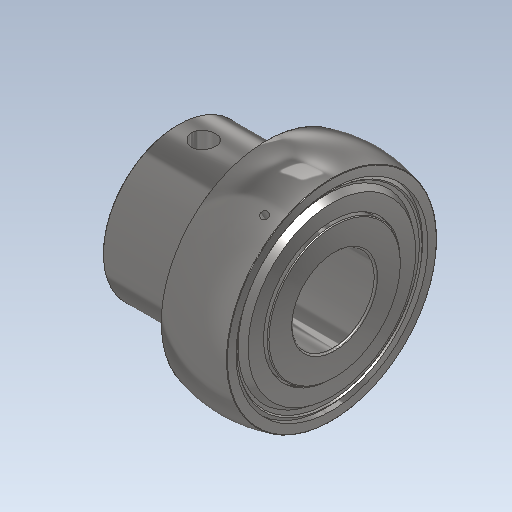
# Autodesk Inventor part: YET 203/15-24.21030112021228.6-bearing
Saved by Autodesk Inventor 2020 (Build 240168000, 168)
## iProperties
Part Number: YET 203/15-24.21030112021228.6-bearing
Material: Stainless Steel
Catalog Web Link: www.cadenas.de
Description: ayf_001hc_hh_hy_bearing-Y-bearings
Vendor: SKF
Document SubType Name: Modeling
Designer: partserver
Manufacturer: SKF
Mass: 107.476 g
Surface Area: 122.39 cm^2
Volume: 13.4345 cm^3
Density: 8 g/cm^3
Appearance: Semi-Polished
Category: PARTsolutions
Company: SKF
PSOL_IDENT_0: {$CADENAS_DATA\23d-libs\skf\bearings_units_and_housings\bearing_units\ball_bearing_units\y-units\y-b
PSOL_IDENT_1: earing_square_flanged_units_parts\ayf_001hc_hh_hy_bearing.prj},235 {VTYP=3D},{NB=YET 203/15-24.21030
PSOL_IDENT_2: 112021228.6-bearing},{LINA=YET 203/15-24.21030112021228.6-bearing},{NN=ayf_001hc_hh_hy_bearing},{DAT
PSOL_IDENT_3: E=20.08.2020 13:45:20},{GEOMDATE=29.07.2020 17:09:33},{VERSION=},{LINEID=2150},{WBVAR=},{WBNUMERIC=}
PSOL_IDENT_4: {NB=YET 203/15-24.21030112021228.6-bearing},{LINA=YET 203/15-24.21030112021228.6-bearing},{KT=DUMM
PSOL_IDENT_5: Y},{PRODUCTID=103011202},{DESIGNATION=YET 203/15},{DD=15.0000},{D=40},{B=19.100},{C=12.000},{PITCH=2
PSOL_IDENT_6: 8.500},{DW=6.747},{FO=IEC_BBY_005},{DESIGN=ybrg2},{B1=28.600},{LM=Eccentric locking collar},{DES=Inn
PSOL_IDENT_7: er ring extended on one side},{PS=For agricultural applications},{MAT=},{SS=Standard seals},{UNIT=Me
PSOL_IDENT_8: tric},{G=MIN},{DD1=24.20},{DD2=27.20},{DD3=MIN},{B3=13.500},{B4=4.8},{BB4=MIN},{R12=0.3},{R12X=0},{S
PSOL_IDENT_9: S1=22.100},{NOTE=},{DG=MIN},{E=3.600},{F=1.300},{RG=MIN},{LOAD1=9.560},{LOAD2=4.750},{LOAD3=0.200},{
PSOL_IDENT_10: SPEED2=9500},{FF0=13},{BF=1},{A15=500000},{A8=400000},{A4=300000},{BETA=1.89},{SBT1=0.094},{SBT2=},{
PSOL_IDENT_11: RF1=0.00000039},{RF2=1.7},{SF1=0.00323},{SF2=36.5},{KZ=3.1},{II=1},{Z=8},{SG=VT307},{MASS=0.12},{G2=
PSOL_IDENT_12: M6x0.75},{HEX=3.000},{RTT=4},{MKIT=},{AS=},{TANGLE=},{SLEEVE=},{SRING=RIS 203},{FPC=RBC17_YBRG_003},
PSOL_IDENT_13: {POPI=1},{NOUN=N020},{NOUNDES=Ball bearing},{MOD=M200},{MODDES=Radial deep groove},{YZ=12.1},{PIM=YE
PSOL_IDENT_14: T 203/15},{LNDD11=MIN},{LUB3=0},{BZ=0.3502},{SDALG=h},{YRZ=17.6235},{SHAPE=1},{LNB1HM11=0},{LWM=0},{
PSOL_IDENT_15: TYPEID=103011},{LUBGR2=0},{LOCKNUT=},{LOCKDEVICE=},{LNB=MIN},{BB=MIN},{LNB1=MIN},{S1ALG=0},{HH=MIN},
PSOL_IDENT_16: {LDB=MIN},{LDDD1=MIN},{LDDD2=MIN},{LDM=MIN},{LDFF=MIN},{TP=4},{LNBHM11=0},{BBHM11=0},{LNDD1HM11=0},{
PSOL_IDENT_17: HELP=3},{HHHM11=0},{LUBGR1=0},{LWV=0},{S2=0},{LUB2=1},{BZ1=0.000},{HEX2=}
NB: YET 203/15-24.21030112021228.6-bearing
NN: ayf_001hc_hh_hy_bearing
NT: Y-bearings
NBSYN: $DESIGNATION.-$DD1.$PRODUCTID.$C.$B1.-bearing
LINA: YET 203/15-24.21030112021228.6-bearing
CATALOG: SKF
DESIGNATION: YET 203/15
DD: 15
D: 40
B: 19.1
C: 12
B1: 28.6
DD1: 24.2
LOAD1: 9.56
LOAD2: 4.75
LOAD3: 0.2
SPEED2: 9500
SUPPLIER: SKF
ARTICLENO: YET 203/15-24.21030112021228.6-bearing
BOMINFO: YET 203/15-24.21030112021228.6-bearing
CREATOR: CADENAS GmbH
Title: YET 203/15-24.21030112021228.6-bearing
Author: Cadenas PARTsolutions
Comments: Y-bearings
Autodesk Inventor part; units mm, degrees
sketch "Sketch_1" plane through (0, 0, 0) normal (0, 0, 1) x (1, 0, 0)
  line L0 (12.3, 0) -> (-6.2, 0)
  arc A0 (-6.5, 7.8) -> (-6.2, 7.5) centre (-6.2, 7.8) ccw
  line L1 (-6.2, 7.5) -> (12.3, 7.5)
  arc A1 (12.3, 7.5) -> (12.6, 7.8) centre (12.3, 7.8) ccw
  line L2 (12.6, 7.8) -> (12.6, 11.45)
  arc A2 (12.6, 11.45) -> (12.45, 11.6) centre (12.45, 11.45) ccw
  line L3 (12.45, 11.6) -> (8.6, 11.6)
  line L4 (8.6, 11.6) -> (8.6, 12.1)
  line L5 (8.6, 12.1) -> (2.5996, 12.1)
  arc A3 (-2.5996, 12.1) -> (2.5996, 12.1) centre (0, 14.25) ccw
  line L6 (-2.5996, 12.1) -> (-6.35, 12.1)
  arc A4 (-6.35, 12.1) -> (-6.5, 11.95) centre (-6.35, 11.95) ccw
  line L7 (-6.5, 11.95) -> (-6.5, 7.8)
  constraints: 16 end point, 10 point on circle, 5 centre point
revolve "Revolution1" add sketch "Sketch_1" angle 360 about axis through (12.3, 0, 0) along (1, 0, 0)
sketch "Sketch_4" plane through (0, 0, 0) normal (0, 0, 1) x (1, 0, 0)
  line L0 (50, 0) -> (-50, 0)
  line L1 (-6, 15.2347) -> (-6, 12.4314)
  line L2 (-6, 12.4314) -> (-5.6498, 12.4314)
  line L3 (-5.6498, 12.4314) -> (-5.6498, 15.0594)
  line L4 (-5.6498, 15.0594) -> (-4.8797, 15.6359)
  line L5 (-4.8797, 15.6359) -> (-4.8377, 15.5798)
  line L6 (-4.8377, 15.5798) -> (-5.5798, 15.0244)
  line L7 (-5.5798, 15.0244) -> (-5.5798, 12.5971)
  line L8 (-5.5798, 12.5971) -> (-4.9611, 12.5971)
  line L9 (-4.9611, 12.5971) -> (-5.0661, 12.1)
  line L10 (-5.0661, 12.1) -> (-4.7159, 12.1)
  line L11 (-4.7159, 12.1) -> (-4.5992, 12.6524)
  line L12 (-4.5992, 12.6524) -> (-4.5992, 13.2047)
  line L13 (-4.5992, 13.2047) -> (-5.0661, 13.757)
  line L14 (-5.0661, 13.757) -> (-5.0661, 14.8618)
  line L15 (-5.0661, 14.8618) -> (-4.5992, 15.4141)
  line L16 (-4.5992, 15.4141) -> (-4.5992, 17.5735)
  arc A0 (-4.5992, 17.5735) -> (-4.6492, 17.6235) centre (-4.6492, 17.5735) ccw
  line L17 (-4.6492, 17.6235) -> (-4.8994, 17.6235)
  arc A1 (-4.8994, 17.6235) -> (-4.9494, 17.5735) centre (-4.8994, 17.5735) ccw
  line L18 (-4.9494, 17.5735) -> (-5.5679, 16.8364)
  line L19 (-5.5679, 16.8364) -> (-5.2996, 16.6113)
  line L20 (-5.2996, 16.6113) -> (-4.9494, 17.0287)
  line L21 (-4.9494, 17.0287) -> (-4.9494, 16.0211)
  line L22 (-4.9494, 16.0211) -> (-6, 15.2347)
  constraints: 46 end point, 4 point on circle, 2 centre point
revolve "Revolution2" add sketch "Sketch_4" angle 360 about axis through (50, 0, 0) along (1, 0, 0)
sketch "Sketch_9" plane through (0, 0, 0) normal (0, 0, 1) x (1, 0, 0)
  line L0 (50, 0) -> (-50, 0)
  line L1 (4.5992, 17.5735) -> (4.5992, 15.4141)
  line L2 (4.5992, 15.4141) -> (5.0661, 14.8618)
  line L3 (5.0661, 14.8618) -> (5.0661, 13.757)
  line L4 (5.0661, 13.757) -> (4.5992, 13.2047)
  line L5 (4.5992, 13.2047) -> (4.5992, 12.6524)
  line L6 (4.5992, 12.6524) -> (4.7159, 12.1)
  line L7 (4.7159, 12.1) -> (5.0661, 12.1)
  line L8 (5.0661, 12.1) -> (4.9611, 12.5971)
  line L9 (4.9611, 12.5971) -> (5.5798, 12.5971)
  line L10 (5.5798, 12.5971) -> (5.5798, 15.0244)
  line L11 (5.5798, 15.0244) -> (4.8377, 15.5798)
  line L12 (4.8377, 15.5798) -> (4.8797, 15.6359)
  line L13 (4.8797, 15.6359) -> (5.6498, 15.0594)
  line L14 (5.6498, 15.0594) -> (5.6498, 12.4314)
  line L15 (5.6498, 12.4314) -> (6, 12.4314)
  line L16 (6, 12.4314) -> (6, 15.2347)
  line L17 (6, 15.2347) -> (4.9494, 16.0211)
  line L18 (4.9494, 16.0211) -> (4.9494, 17.0287)
  line L19 (4.9494, 17.0287) -> (5.2996, 16.6113)
  line L20 (5.2996, 16.6113) -> (5.5679, 16.8364)
  line L21 (5.5679, 16.8364) -> (4.9494, 17.5735)
  arc A0 (4.9494, 17.5735) -> (4.8994, 17.6235) centre (4.8994, 17.5735) ccw
  line L22 (4.8994, 17.6235) -> (4.6492, 17.6235)
  arc A1 (4.6492, 17.6235) -> (4.5992, 17.5735) centre (4.6492, 17.5735) ccw
  constraints: 46 end point, 4 point on circle, 2 centre point
revolve "Revolution3" add sketch "Sketch_9" angle 360 about axis through (50, 0, 0) along (1, 0, 0)
sketch "Sketch_14" plane through (0, 0, 0) normal (0, 0, 1) x (1, 0, 0)
  line L0 (6, 0) -> (-6, 0)
  line L1 (-6, 17.4484) -> (-5.0228, 17.4484)
  line L2 (-5.0228, 17.4484) -> (-4.9192, 17.5251)
  arc A0 (-4.5686, 17.44) -> (-4.9192, 17.5251) centre (-4.7643, 17.3984) ccw
  line L3 (-4.5686, 17.44) -> (-4.4641, 16.9488)
  line L4 (-4.4641, 16.9488) -> (-2.0241, 16.9488)
  arc A1 (2.0241, 16.9488) -> (-2.0241, 16.9488) centre (0, 14.25) ccw
  line L5 (2.0241, 16.9488) -> (4.4641, 16.9488)
  line L6 (4.4641, 16.9488) -> (4.5686, 17.44)
  arc A2 (4.8889, 17.5549) -> (4.5686, 17.44) centre (4.7643, 17.3984) ccw
  line L7 (4.8889, 17.5549) -> (5.0228, 17.4484)
  line L8 (5.0228, 17.4484) -> (6, 17.4484)
  line L9 (6, 17.4484) -> (6, 19.0053)
  arc A3 (6, 19.0053) -> (5.9296, 19.1008) centre (5.9, 19.0053) ccw
  arc A4 (5.9296, 19.1008) -> (-5.9296, 19.1008) centre (0, 0) ccw
  arc A5 (-5.9296, 19.1008) -> (-6, 19.0053) centre (-5.9, 19.0053) ccw
  line L10 (-6, 19.0053) -> (-6, 17.4484)
  constraints: 22 end point, 12 point on circle, 6 centre point
revolve "Revolution4" add sketch "Sketch_14" angle 360 about axis through (6, 0, 0) along (1, 0, 0)
sketch "Sketch_15" plane through (0, 0, 0) normal (0, 0, 1) x (1, 0, 0)
  line L0 (-2.1, 21) -> (-2.1, 14.25)
  line L1 (-2.1, 14.25) -> (-2.75, 14.25)
  line L2 (-2.75, 14.25) -> (-2.75, 21)
  line L3 (-2.75, 21) -> (-2.1, 21)
  line L4 (-2.1, 21) -> (-2.1, 14.25)
  constraints: 10 end point
revolve "Revolution5" cut sketch "Sketch_15" angle 360 about axis through (-2.1, 21, 0) along (0, 1, 0)
sketch "Sketch_16" plane through (0, 0, 0) normal (0, 0.8660254, -0.5) x (1, 0, 0)
  line L0 (-3.6, 21) -> (-3.6, 14.25)
  line L1 (-3.6, 14.25) -> (-4.25, 14.25)
  line L2 (-4.25, 14.25) -> (-4.25, 21)
  line L3 (-4.25, 21) -> (-3.6, 21)
  line L4 (-3.6, 21) -> (-3.6, 14.25)
  constraints: 10 end point
revolve "Revolution6" cut sketch "Sketch_16" angle 360 about axis through (-3.6, -10.5, -18.1865) along (0, -0.5, -0.8660254)
sketch "Sketch_17" plane through (0, 0, 0) normal (0, 0, 1) x (1, 0, 0)
  line L0 (21.8, 0) -> (12.9, 0)
  line L1 (8.6, 13.3) -> (8.6, 12.25)
  line L2 (8.6, 12.25) -> (8.75, 12.1)
  line L3 (8.75, 12.1) -> (12.6, 12.1)
  line L4 (12.6, 12.1) -> (12.6, 7.8)
  line L5 (12.6, 7.8) -> (12.9, 7.5)
  line L6 (12.9, 7.5) -> (21.8, 7.5)
  line L7 (21.8, 7.5) -> (22.1, 7.8)
  line L8 (22.1, 7.8) -> (22.1, 13.45)
  arc A0 (22.1, 13.45) -> (21.95, 13.6) centre (21.95, 13.45) ccw
  line L9 (21.95, 13.6) -> (8.9, 13.6)
  arc A1 (8.9, 13.6) -> (8.6, 13.3) centre (8.9, 13.3) ccw
  constraints: 20 end point, 4 point on circle, 2 centre point
revolve "Revolution7" add sketch "Sketch_17" angle 360 about axis through (21.8, 0, 0) along (1, 0, 0)
sketch "Sketch_18" plane through (0, 0, 0) normal (0, 0, 1) x (1, 0, 0)
  line L0 (17.3, 7.5) -> (17.3, 13.905)
  line L1 (17.3, 13.905) -> (20.3, 13.905)
  line L2 (20.3, 13.905) -> (20.3, 7.5)
  line L3 (20.3, 7.5) -> (17.3, 7.5)
  line L4 (17.3, 7.5) -> (17.3, 13.905)
  constraints: 10 end point
revolve "Revolution8" add sketch "Sketch_18" angle 360 about axis through (17.3, 7.5, 0) along (0, -1, 0)
sketch "Sketch_19" plane through (17.3, 13.905, 0) normal (0, 1, 0) x (1, 0, 0)
  line L0 (-1.5, -0.866) -> (0, -1.7321)
  line L1 (0, -1.7321) -> (1.5, -0.866)
  line L2 (1.5, -0.866) -> (1.5, 0.866)
  line L3 (1.5, 0.866) -> (0, 1.7321)
  line L4 (0, 1.7321) -> (-1.5, 0.866)
  line L5 (-1.5, 0.866) -> (-1.5, -0.866)
  constraints: 12 end point
extrude "Extrusion1" cut sketch "Sketch_19" against normal blind 0.61
sketch "Sketch_20" plane through (0, 0, 0) normal (0, 1, 0) x (-1, 0, 0)
  line L0 (-17.3, -9.3029) -> (-17.3, -13.905)
  line L1 (-17.3, -13.905) -> (-19.46, -13.905)
  line L2 (-19.46, -13.905) -> (-19.46, -10.55)
  line L3 (-19.46, -10.55) -> (-17.3, -9.3029)
  line L4 (-17.3, -9.3029) -> (-17.3, -13.905)
  constraints: 10 end point
revolve "Revolution9" cut sketch "Sketch_20" angle 360 about axis through (17.3, 0, -9.3029) along (0, 0, 1)
ref_plane "ball_1_XY" through (0, 14.25, 0) normal (1, 0, 0) x (0, 0, -1)
ref_plane "ball_1_YZ" through (0, 14.25, 0) normal (0, 0, -1) x (0, 1, 0)
ref_plane "ball_1_ZX" through (0, 14.25, 0) normal (0, 1, 0) x (1, 0, 0)
ref_plane "ball_2_XY" through (0, 10.0763, 10.0763) normal (1, 0, 0) x (0, 0, -1)
ref_plane "ball_2_YZ" through (0, 10.0763, 10.0763) normal (0, 0, -1) x (0, 1, 0)
ref_plane "ball_2_ZX" through (0, 10.0763, 10.0763) normal (0, 1, 0) x (1, 0, 0)
ref_plane "ball_3_XY" through (0, 0, 14.25) normal (1, 0, 0) x (0, 0, -1)
ref_plane "ball_3_YZ" through (0, 0, 14.25) normal (0, 0, -1) x (0, 1, 0)
ref_plane "ball_3_ZX" through (0, 0, 14.25) normal (0, 1, 0) x (1, 0, 0)
ref_plane "ball_4_XY" through (0, -10.0763, 10.0763) normal (1, 0, 0) x (0, 0, -1)
ref_plane "ball_4_YZ" through (0, -10.0763, 10.0763) normal (0, 0, -1) x (0, 1, 0)
ref_plane "ball_4_ZX" through (0, -10.0763, 10.0763) normal (0, 1, 0) x (1, 0, 0)
ref_plane "ball_5_XY" through (0, -14.25, 0) normal (1, 0, 0) x (0, 0, -1)
ref_plane "ball_5_YZ" through (0, -14.25, 0) normal (0, 0, -1) x (0, 1, 0)
ref_plane "ball_5_ZX" through (0, -14.25, 0) normal (0, 1, 0) x (1, 0, 0)
ref_plane "ball_6_XY" through (0, -10.0763, -10.0763) normal (1, 0, 0) x (0, 0, -1)
ref_plane "ball_6_YZ" through (0, -10.0763, -10.0763) normal (0, 0, -1) x (0, 1, 0)
ref_plane "ball_6_ZX" through (0, -10.0763, -10.0763) normal (0, 1, 0) x (1, 0, 0)
ref_plane "ball_7_XY" through (0, 0, -14.25) normal (1, 0, 0) x (0, 0, -1)
ref_plane "ball_7_YZ" through (0, 0, -14.25) normal (0, 0, -1) x (0, 1, 0)
ref_plane "ball_7_ZX" through (0, 0, -14.25) normal (0, 1, 0) x (1, 0, 0)
ref_plane "ball_8_XY" through (0, 10.0763, -10.0763) normal (1, 0, 0) x (0, 0, -1)
ref_plane "ball_8_YZ" through (0, 10.0763, -10.0763) normal (0, 0, -1) x (0, 1, 0)
ref_plane "ball_8_ZX" through (0, 10.0763, -10.0763) normal (0, 1, 0) x (1, 0, 0)
ref_plane "brg_XY" through (0, 0, 0) normal (1, 0, 0) x (0, 0, -1)
ref_plane "brg_YZ" through (0, 0, 0) normal (0, 0, -1) x (0, 1, 0)
ref_plane "brg_ZX" through (0, 0, 0) normal (0, 1, 0) x (1, 0, 0)
ref_plane "brg3_XY" through (22.1, 0, 0) normal (1, 0, 0) x (0, 0, -1)
ref_plane "brg3_YZ" through (22.1, 0, 0) normal (0, 0, -1) x (0, 1, 0)
ref_plane "brg3_ZX" through (22.1, 0, 0) normal (0, 1, 0) x (1, 0, 0)
body "Solid1"
